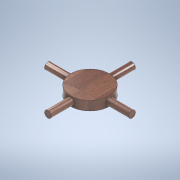
# Autodesk Inventor part: CapMid-ver1-1111-2021
Saved by Autodesk Inventor 2021 (Build 250183000, 183)
## iProperties
Created: 2021-03-03
Part Number: CapMid-ver1-1111-2021
Material: Generic
Document SubType Name: Modeling
Designer: CMurray
Density: 1 g/cm^3
Appearance: Default
Author: CMurray
Autodesk Inventor part; units mm, degrees
sketch "Sketch1" plane through (0, 0, 0) normal (0, 1, 0) x (-1, 0, 0)
  circle A0 centre (0, 0) radius 107.95
  dimension "d0" = 215.9
  constraints: 1 centre point, 1 coincident
  measures "d0" diameter of A0
extrude "Extrusion1" add sketch "Sketch1" along normal blind 50.8
ref_plane "Work Plane1" through (0, 25.4, 0) normal (0, 1, 0) x (1, 0, 0)
ref_plane "Work Plane3" through (107.95, 0, 0) normal (-1, 0, 0) x (0, -1, 0)
ref_plane "Work Plane2" through (-107.95, 0, 0) normal (-1, 0, 0) x (0, -1, 0)
ref_plane "Work Plane5" through (0, 0, -107.95) normal (0, 0, 1) x (1, 0, 0)
ref_plane "Work Plane4" through (0, 0, 107.95) normal (0, 0, 1) x (1, 0, 0)
sketch "Sketch4" plane through (0, 0, -107.95) normal (0, 0, 1) x (1, 0, 0)
  circle A0 centre (0, 25.4) radius 19.05
  line L0 (107.95, 0) -> (-107.95, 0) projected
  point P0 (0, 0)
  dimension "d9" = 38.1
  dimension "d10" = 25.4
  constraints: 1 centre point
  measures "d9" diameter of A0
  measures "d10" distance from line of L0 A0.centre
extrude "Extrusion4" add sketch "Sketch4" against normal blind 127
sketch "Sketch5" plane through (-107.95, 0, 0) normal (-1, 0, 0) x (0, -1, 0)
  circle A0 centre (-25.4, 0) radius 19.05
  line L0 (0, 107.95) -> (0, -107.95) projected
  point P0 (0, 0)
  dimension "d13" = 38.1
  dimension "d14" = 25.4
  constraints: 1 centre point
  measures "d13" diameter of A0
  measures "d14" distance from line of L0 A0.centre
extrude "Extrusion5" add sketch "Sketch5" along normal blind 127
sketch "Sketch6" plane through (0, 0, 107.95) normal (0, 0, 1) x (1, 0, 0)
  line L0 (0, 6.35) -> (0, 44.45) projected
  circle A0 centre (0, 25.4) radius 19.05
  point P0 (0, 0)
  constraints: 1 centre point, 1 midpoint
extrude "Extrusion6" add sketch "Sketch6" along normal blind 127
sketch "Sketch7" plane through (107.95, 0, 0) normal (-1, 0, 0) x (0, -1, 0)
  arc A0 (-6.35, 0) -> (-44.45, 0) centre (-25.4, 0) ccw projected
  circle A1 centre (-25.4, 0) radius 19.05
  point P0 (0, 0)
  point P1 (-6.35, 0)
  constraints: 1 centre point, 1 coincident
extrude "Extrusion7" add sketch "Sketch7" against normal blind 127
body "Solid1"
